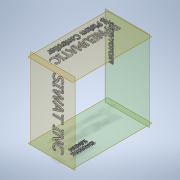
# Autodesk Inventor part: BaseTextYellow
Saved by Autodesk Inventor 2022.2 (Build 262287000, 287)
## iProperties
Created: 2022-01-15
Part Number: BaseTextYellow
Material: Generic
Document SubType Name: Modeling
Designer: siwat
Density: 1 g/cm^3
Appearance: Default
Author: siwat
Autodesk Inventor part; units mm, degrees
(part 1 of 2)
ref_plane "YZ Plane" through (0, 0, 0) normal (1, 0, 0) x (0, 1, 0)
ref_plane "XZ Plane" through (0, 0, 0) normal (0, 1, 0) x (-1, 0, 0)
ref_plane "XY Plane" through (0, 0, 0) normal (0, 0, 1) x (1, 0, 0)
ref_plane "Work Plane1" through (0, 0, 0) normal (0, 0, 1) x (1, 0, 0)
sketch "Sketch1" plane through (0, 0, 0) normal (0, 0, 1) x (1, 0, 0)
  line L0 (54.655, -7.723) -> (54.655, -141.093) construction
  line L1 (54.655, -141.093) -> (34.3574, -141.093) construction
  line L2 (34.3574, -141.093) -> (34.3574, -7.723) construction
  line L3 (34.3574, -7.723) -> (54.655, -7.723) construction
  spline S0 degree 2 poles (34.9775, -14.9442) (34.9775, -12.881) (35.8397, -9.9864) (36.4556, -8.7084) knots 0 0 0 1 2 2 2
  line L4 (36.4556, -8.7084) -> (39.6274, -8.7084)
  line L5 (39.6274, -8.7084) -> (39.6274, -8.8932)
  spline S1 degree 2 poles (39.6274, -8.8932) (38.4572, -10.1403) (37.1639, -13.2967) (37.1639, -14.7594) knots 0 0 0 1 2 2 2
  spline S2 degree 2 poles (37.1639, -14.7594) (37.1639, -16.8535) (38.9037, -18.9936) (40.3357, -18.9936) knots 0 0 0 1 2 2 2
  spline S3 degree 2 poles (40.3357, -18.9936) (41.4751, -18.9936) (42.8916, -17.8697) (43.2457, -16.6533) knots 0 0 0 1 2 2 2
  spline S4 degree 2 poles (43.2457, -16.6533) (43.4921, -15.7757) (43.8308, -14.3129) (44.108, -13.2197) knots 0 0 0 1 2 2 2
  spline S5 degree 2 poles (44.108, -13.2197) (44.3697, -12.2343) (45.155, -10.6792) (45.7862, -10.0787) knots 0 0 0 1 2 2 2
  spline S6 degree 2 poles (45.7862, -10.0787) (46.4175, -9.4936) (48.1112, -8.847) (49.2198, -8.847) knots 0 0 0 1 2 2 2
  spline S7 degree 2 poles (49.2198, -8.847) (51.5294, -8.847) (54.655, -12.4499) (54.655, -15.2368) knots 0 0 0 1 2 2 2
  spline S8 degree 2 poles (54.655, -15.2368) (54.655, -16.8381) (54.0237, -19.6711) (53.4232, -20.8875) knots 0 0 0 1 2 2 2
  line L6 (53.4232, -20.8875) -> (50.4054, -20.8875)
  line L7 (50.4054, -20.8875) -> (50.4054, -20.7027)
  spline S9 degree 2 poles (50.4054, -20.7027) (51.2368, -19.7943) (52.4686, -16.9612) (52.4686, -15.4061) knots 0 0 0 1 2 2 2
  spline S10 degree 2 poles (52.4686, -15.4061) (52.4686, -13.6509) (50.8211, -11.4799) (49.4815, -11.4799) knots 0 0 0 1 2 2 2
  spline S11 degree 2 poles (49.4815, -11.4799) (48.2806, -11.4799) (46.8486, -12.7578) (46.5253, -13.9588) knots 0 0 0 1 2 2 2
  spline S12 degree 2 poles (46.5253, -13.9588) (46.3097, -14.7594) (45.7554, -17.0844) (45.5245, -17.8543) knots 0 0 0 1 2 2 2
  spline S13 degree 2 poles (45.5245, -17.8543) (44.924, -19.8097) (42.5067, -21.6265) (40.736, -21.6265) knots 0 0 0 1 2 2 2
  spline S14 degree 2 poles (40.736, -21.6265) (39.612, -21.6265) (37.4564, -20.7181) (36.702, -19.9021) knots 0 0 0 1 2 2 2
  spline S15 degree 2 poles (36.702, -19.9021) (35.8705, -18.9936) (34.9775, -16.6841) (34.9775, -14.9442) knots 0 0 0 1 2 2 2
  line L8 (35.3162, -30.8186) -> (35.3162, -23.4588)
  line L9 (35.3162, -23.4588) -> (37.2563, -23.4588)
  line L10 (37.2563, -23.4588) -> (37.2563, -25.8761)
  line L11 (37.2563, -25.8761) -> (52.3762, -25.8761)
  line L12 (52.3762, -25.8761) -> (52.3762, -23.4588)
  line L13 (52.3762, -23.4588) -> (54.3162, -23.4588)
  line L14 (54.3162, -23.4588) -> (54.3162, -30.8186)
  line L15 (54.3162, -30.8186) -> (52.3762, -30.8186)
  line L16 (52.3762, -30.8186) -> (52.3762, -28.4013)
  line L17 (52.3762, -28.4013) -> (37.2563, -28.4013)
  line L18 (37.2563, -28.4013) -> (37.2563, -30.8186)
  line L19 (37.2563, -30.8186) -> (35.3162, -30.8186)
  line L20 (54.3162, -55.2384) -> (35.3162, -50.4653)
  line L21 (35.3162, -50.4653) -> (35.3162, -47.6322)
  line L22 (35.3162, -47.6322) -> (51.0828, -43.7676)
  line L23 (51.0828, -43.7676) -> (35.3162, -40.0107)
  line L24 (35.3162, -40.0107) -> (35.3162, -37.2084)
  line L25 (35.3162, -37.2084) -> (54.3162, -32.3583)
  line L26 (54.3162, -32.3583) -> (54.3162, -34.9604)
  line L27 (54.3162, -34.9604) -> (38.565, -38.7789)
  line L28 (38.565, -38.7789) -> (54.3162, -42.5666)
  line L29 (54.3162, -42.5666) -> (54.3162, -45.1379)
  line L30 (54.3162, -45.1379) -> (38.3802, -48.9564)
  line L31 (38.3802, -48.9564) -> (54.3162, -52.7594)
  line L32 (54.3162, -52.7594) -> (54.3162, -55.2384)
  line L33 (35.3162, -55.4539) -> (54.3162, -61.8591)
  line L34 (54.3162, -61.8591) -> (54.3162, -64.9693)
  line L35 (54.3162, -64.9693) -> (35.3162, -71.3745)
  line L36 (35.3162, -71.3745) -> (35.3162, -68.7108)
  line L37 (35.3162, -68.7108) -> (40.6282, -66.9864)
  line L38 (40.6282, -66.9864) -> (40.6282, -59.7343)
  line L39 (40.6282, -59.7343) -> (35.3162, -58.0099)
  line L40 (35.3162, -58.0099) -> (35.3162, -55.4539)
  line L41 (42.7838, -66.2935) -> (51.7295, -63.3526)
  line L42 (51.7295, -63.3526) -> (42.7838, -60.4272)
  line L43 (42.7838, -60.4272) -> (42.7838, -66.2935)
  line L44 (35.3162, -77.6103) -> (52.0683, -77.6103)
  line L45 (52.0683, -77.6103) -> (52.0683, -71.2359)
  line L46 (52.0683, -71.2359) -> (54.3162, -71.2359)
  line L47 (54.3162, -71.2359) -> (54.3162, -86.5099)
  line L48 (54.3162, -86.5099) -> (52.0683, -86.5099)
  line L49 (52.0683, -86.5099) -> (52.0683, -80.1355)
  line L50 (52.0683, -80.1355) -> (35.3162, -80.1355)
  line L51 (35.3162, -80.1355) -> (35.3162, -77.6103)
  line L52 (35.3162, -103.2157) -> (35.3162, -95.8559)
  line L53 (35.3162, -95.8559) -> (37.2563, -95.8559)
  line L54 (37.2563, -95.8559) -> (37.2563, -98.2732)
  line L55 (37.2563, -98.2732) -> (52.3762, -98.2732)
  line L56 (52.3762, -98.2732) -> (52.3762, -95.8559)
  line L57 (52.3762, -95.8559) -> (54.3162, -95.8559)
  line L58 (54.3162, -95.8559) -> (54.3162, -103.2157)
  line L59 (54.3162, -103.2157) -> (52.3762, -103.2157)
  line L60 (52.3762, -103.2157) -> (52.3762, -100.7983)
  line L61 (52.3762, -100.7983) -> (37.2563, -100.7983)
  line L62 (37.2563, -100.7983) -> (37.2563, -103.2157)
  line L63 (37.2563, -103.2157) -> (35.3162, -103.2157)
  line L64 (35.3162, -119.9369) -> (35.3162, -117.1039)
  line L65 (35.3162, -117.1039) -> (51.6987, -108.697)
  line L66 (51.6987, -108.697) -> (35.3162, -108.697)
  line L67 (35.3162, -108.697) -> (35.3162, -106.3413)
  line L68 (35.3162, -106.3413) -> (54.3162, -106.3413)
  line L69 (54.3162, -106.3413) -> (54.3162, -109.9288)
  line L70 (54.3162, -109.9288) -> (39.2733, -117.5812)
  line L71 (39.2733, -117.5812) -> (54.3162, -117.5812)
  line L72 (54.3162, -117.5812) -> (54.3162, -119.9369)
  line L73 (54.3162, -119.9369) -> (35.3162, -119.9369)
  spline S16 degree 2 poles (34.9775, -131.2076) (34.9775, -129.3599) (36.2247, -126.2343) (37.4718, -125.0949) knots 0 0 0 1 2 2 2
  spline S17 degree 2 poles (37.4718, -125.0949) (38.7036, -123.9556) (42.3989, -122.7084) (44.8008, -122.7084) knots 0 0 0 1 2 2 2
  spline S18 degree 2 poles (44.8008, -122.7084) (47.1874, -122.7084) (50.7287, -123.9248) (52.0375, -125.0795) knots 0 0 0 1 2 2 2
  spline S19 degree 2 poles (52.0375, -125.0795) (53.3154, -126.2189) (54.655, -129.3291) (54.655, -131.2538) knots 0 0 0 1 2 2 2
  spline S20 degree 2 poles (54.655, -131.2538) (54.655, -132.2084) (54.3778, -133.8867) (54.1623, -134.5949) knots 0 0 0 1 2 2 2
  spline S21 degree 2 poles (54.1623, -134.5949) (53.9621, -135.2108) (53.3924, -136.4888) (53.0537, -137.1201) knots 0 0 0 1 2 2 2
  line L74 (53.0537, -137.1201) -> (50.005, -137.1201)
  line L75 (50.005, -137.1201) -> (50.005, -136.9199)
  spline S22 degree 2 poles (50.005, -136.9199) (50.313, -136.5812) (51.1752, -135.5342) (51.5909, -134.7797) knots 0 0 0 1 2 2 2
  spline S23 degree 2 poles (51.5909, -134.7797) (51.9913, -134.056) (52.4994, -132.347) (52.4994, -131.2384) knots 0 0 0 1 2 2 2
  spline S24 degree 2 poles (52.4994, -131.2384) (52.4994, -130.022) (51.4986, -127.851) (50.5439, -127.035) knots 0 0 0 1 2 2 2
  spline S25 degree 2 poles (50.5439, -127.035) (49.5739, -126.2343) (46.6331, -125.3413) (44.8008, -125.3413) knots 0 0 0 1 2 2 2
  spline S26 degree 2 poles (44.8008, -125.3413) (42.8454, -125.3413) (40.0277, -126.2805) (39.0577, -127.0966) knots 0 0 0 1 2 2 2
  spline S27 degree 2 poles (39.0577, -127.0966) (38.1185, -127.8972) (37.1639, -130.0374) (37.1639, -131.2384) knots 0 0 0 1 2 2 2
  spline S28 degree 2 poles (37.1639, -131.2384) (37.1639, -132.3316) (37.7028, -134.1946) (38.1031, -134.9183) knots 0 0 0 1 2 2 2
  spline S29 degree 2 poles (38.1031, -134.9183) (38.5034, -135.6111) (39.3349, -136.6428) (39.6274, -136.9353) knots 0 0 0 1 2 2 2
  line L76 (39.6274, -136.9353) -> (39.6274, -137.1201)
  line L77 (39.6274, -137.1201) -> (36.6096, -137.1201)
  spline S30 degree 2 poles (36.6096, -137.1201) (36.317, -136.4888) (35.7781, -135.3802) (35.5318, -134.5949) knots 0 0 0 1 2 2 2
  spline S31 degree 2 poles (35.5318, -134.5949) (35.2546, -133.7635) (34.9775, -132.347) (34.9775, -131.2076) knots 0 0 0 1 2 2 2
  point P0 (0, 0)
  constraints: 2 other
extrude "Extrusion1" add sketch "Sketch1" against normal blind 2
ref_plane "Work Plane2" through (0, 0, -142.4319) normal (0.0000018, 1, 0) x (0.0015858, 0, 0.9999987)
sketch "Sketch2" plane through (0, 0, -142.4319) normal (0.0000018, 1, 0) x (0.0015858, 0, 0.9999987)
  line L0 (22.3492, 32.6802) -> (316.1985, 32.6802) construction
  line L1 (316.1985, 32.6802) -> (316.1985, 7.1194) construction
  line L2 (316.1985, 7.1194) -> (22.3492, 7.1194) construction
  line L3 (22.3492, 7.1194) -> (22.3492, 32.6802) construction
  line L4 (22.2144, 12.4409) -> (316.0637, 12.4409) construction
  line L5 (316.0637, 12.4409) -> (316.0637, -3.1912) construction
  line L6 (316.0637, -3.1912) -> (22.2144, -3.1912) construction
  line L7 (22.2144, -3.1912) -> (22.2144, 12.4409) construction
  line L8 (10.9639, 9.125) -> (10.9639, 34.4309) construction
  line L9 (10.9639, 34.4309) -> (304.8132, 34.4309) construction
  line L10 (304.8132, 34.4309) -> (304.8132, 9.125) construction
  line L11 (304.8132, 9.125) -> (10.9639, 9.125) construction
  spline S0 degree 2 poles (19.8618, 29.4228) (19.8618, 28.0533) (18.7516, 25.8491) (17.8197, 25.2332) knots 0 0 0 1 2 2 2
  spline S1 degree 2 poles (17.8197, 25.2332) (17.0579, 24.7551) (15.4939, 24.4309) (14.2784, 24.4309) knots 0 0 0 1 2 2 2
  line L12 (14.2784, 24.4309) -> (11.9769, 24.4309)
  line L13 (11.9769, 24.4309) -> (11.9769, 34.4309)
  line L14 (11.9769, 34.4309) -> (14.254, 34.4309)
  spline S2 degree 2 poles (14.254, 34.4309) (15.6641, 34.4309) (17.2686, 34.0096) (17.8359, 33.6368) knots 0 0 0 1 2 2 2
  spline S3 degree 2 poles (17.8359, 33.6368) (18.8002, 32.9966) (19.8618, 30.8815) (19.8618, 29.4228) knots 0 0 0 1 2 2 2
  spline S4 degree 2 poles (18.4761, 29.439) (18.4761, 30.5898) (17.7143, 32.2186) (16.9607, 32.6805) knots 0 0 0 1 2 2 2
  spline S5 degree 2 poles (16.9607, 32.6805) (16.4258, 32.9966) (15.2184, 33.2802) (14.3189, 33.2802) knots 0 0 0 1 2 2 2
  line L15 (14.3189, 33.2802) -> (13.3059, 33.2802)
  line L16 (13.3059, 33.2802) -> (13.3059, 25.5817)
  line L17 (13.3059, 25.5817) -> (14.3189, 25.5817)
  spline S6 degree 2 poles (14.3189, 25.5817) (15.2022, 25.5817) (16.5393, 25.8653) (17.0823, 26.2462) knots 0 0 0 1 2 2 2
  spline S7 degree 2 poles (17.0823, 26.2462) (17.7792, 26.7162) (18.4761, 28.2721) (18.4761, 29.439) knots 0 0 0 1 2 2 2
  line L18 (17.8602, 12.4309) -> (11.6933, 12.4309)
  line L19 (11.6933, 12.4309) -> (11.6933, 13.8491)
  spline S8 degree 2 poles (11.6933, 13.8491) (12.3578, 14.4731) (13.5409, 15.6319) (14.1082, 16.2559) knots 0 0 0 1 2 2 2
  spline S9 degree 2 poles (14.1082, 16.2559) (15.2508, 17.512) (16.0855, 19.0193) (16.0855, 19.8215) knots 0 0 0 1 2 2 2
  spline S10 degree 2 poles (16.0855, 19.8215) (16.0855, 20.2429) (15.8262, 20.875) (15.5912, 21.0776) knots 0 0 0 1 2 2 2
  spline S11 degree 2 poles (15.5912, 21.0776) (15.3562, 21.2802) (14.7403, 21.4828) (14.3675, 21.4828) knots 0 0 0 1 2 2 2
  spline S12 degree 2 poles (14.3675, 21.4828) (14.0109, 21.4828) (13.2816, 21.3045) (12.9493, 21.1668) knots 0 0 0 1 2 2 2
  spline S13 degree 2 poles (12.9493, 21.1668) (12.6657, 21.0533) (12.139, 20.7292) (11.9769, 20.6157) knots 0 0 0 1 2 2 2
  line L20 (11.9769, 20.6157) -> (11.904, 20.6157)
  line L21 (11.904, 20.6157) -> (11.904, 22.042)
  spline S14 degree 2 poles (11.904, 22.042) (12.3173, 22.2446) (13.8002, 22.6416) (14.4647, 22.6416) knots 0 0 0 1 2 2 2
  spline S15 degree 2 poles (14.4647, 22.6416) (15.8667, 22.6416) (17.4469, 21.1587) (17.4469, 19.8945) knots 0 0 0 1 2 2 2
  spline S16 degree 2 poles (17.4469, 19.8945) (17.4469, 19.3029) (17.1714, 18.3143) (16.9283, 17.8929) knots 0 0 0 1 2 2 2
  spline S17 degree 2 poles (16.9283, 17.8929) (16.6852, 17.4553) (15.9801, 16.5963) (15.5912, 16.183) knots 0 0 0 1 2 2 2
  spline S18 degree 2 poles (15.5912, 16.183) (14.9591, 15.4942) (13.4113, 14.0193) (12.9493, 13.5898) knots 0 0 0 1 2 2 2
  line L22 (12.9493, 13.5898) -> (17.8602, 13.5898)
  line L23 (17.8602, 13.5898) -> (17.8602, 12.4309)
  spline S19 degree 2 poles (14.7646, 0.2527) (13.6787, 0.2527) (12.1552, 0.7065) (11.4826, 1.0306) knots 0 0 0 1 2 2 2
  line L24 (11.4826, 1.0306) -> (11.4826, 2.7)
  line L25 (11.4826, 2.7) -> (11.5798, 2.7)
  spline S20 degree 2 poles (11.5798, 2.7) (12.2362, 2.0841) (13.8975, 1.4034) (14.6673, 1.4034) knots 0 0 0 1 2 2 2
  spline S21 degree 2 poles (14.6673, 1.4034) (15.7694, 1.4034) (16.8959, 2.3191) (16.8959, 3.0728) knots 0 0 0 1 2 2 2
  spline S22 degree 2 poles (16.8959, 3.0728) (16.8959, 3.6724) (16.3043, 4.418) (15.6641, 4.6044) knots 0 0 0 1 2 2 2
  spline S23 degree 2 poles (15.6641, 4.6044) (15.2022, 4.734) (14.4323, 4.9123) (13.857, 5.0582) knots 0 0 0 1 2 2 2
  spline S24 degree 2 poles (13.857, 5.0582) (13.3383, 5.1959) (12.5199, 5.6092) (12.2038, 5.9415) knots 0 0 0 1 2 2 2
  spline S25 degree 2 poles (12.2038, 5.9415) (11.8959, 6.2737) (11.5555, 7.1651) (11.5555, 7.7486) knots 0 0 0 1 2 2 2
  spline S26 degree 2 poles (11.5555, 7.7486) (11.5555, 8.9642) (13.4518, 10.6092) (14.9186, 10.6092) knots 0 0 0 1 2 2 2
  spline S27 degree 2 poles (14.9186, 10.6092) (15.7613, 10.6092) (17.2524, 10.277) (17.8926, 9.9609) knots 0 0 0 1 2 2 2
  line L26 (17.8926, 9.9609) -> (17.8926, 8.3726)
  line L27 (17.8926, 8.3726) -> (17.7954, 8.3726)
  spline S28 degree 2 poles (17.7954, 8.3726) (17.3173, 8.8102) (15.8262, 9.4585) (15.0077, 9.4585) knots 0 0 0 1 2 2 2
  spline S29 degree 2 poles (15.0077, 9.4585) (14.0839, 9.4585) (12.9412, 8.5914) (12.9412, 7.8864) knots 0 0 0 1 2 2 2
  spline S30 degree 2 poles (12.9412, 7.8864) (12.9412, 7.2543) (13.6139, 6.5006) (14.2459, 6.3305) knots 0 0 0 1 2 2 2
  spline S31 degree 2 poles (14.2459, 6.3305) (14.6673, 6.217) (15.891, 5.9253) (16.2962, 5.8037) knots 0 0 0 1 2 2 2
  spline S32 degree 2 poles (16.2962, 5.8037) (17.3254, 5.4877) (18.2816, 4.2154) (18.2816, 3.2835) knots 0 0 0 1 2 2 2
  spline S33 degree 2 poles (18.2816, 3.2835) (18.2816, 2.6919) (17.8035, 1.5574) (17.374, 1.1603) knots 0 0 0 1 2 2 2
  spline S34 degree 2 poles (17.374, 1.1603) (16.8959, 0.7227) (15.6803, 0.2527) (14.7646, 0.2527) knots 0 0 0 1 2 2 2
  spline S35 degree 2 poles (33.35, 27.8909) (33.35, 26.9184) (32.6571, 25.168) (32.0372, 24.5602) knots 0 0 0 1 2 2 2
  spline S36 degree 2 poles (32.0372, 24.5602) (31.2592, 23.7944) (29.1563, 23.0043) (27.5518, 23.0043) knots 0 0 0 1 2 2 2
  line L28 (27.5518, 23.0043) -> (25.8621, 23.0043)
  line L29 (25.8621, 23.0043) -> (25.8621, 17.4127)
  line L30 (25.8621, 17.4127) -> (23.8686, 17.4127)
  line L31 (23.8686, 17.4127) -> (23.8686, 32.4127)
  line L32 (23.8686, 32.4127) -> (27.6369, 32.4127)
  spline S37 degree 2 poles (27.6369, 32.4127) (28.974, 32.4127) (30.8459, 31.9751) (31.5631, 31.4768) knots 0 0 0 1 2 2 2
  spline S38 degree 2 poles (31.5631, 31.4768) (32.4019, 30.9055) (33.35, 29.1429) (33.35, 27.8909) knots 0 0 0 1 2 2 2
  spline S39 degree 2 poles (31.2714, 27.8301) (31.2714, 28.608) (30.7365, 29.7507) (30.1895, 30.1153) knots 0 0 0 1 2 2 2
  spline S40 degree 2 poles (30.1895, 30.1153) (29.7155, 30.4314) (28.4513, 30.6867) (27.5153, 30.6867) knots 0 0 0 1 2 2 2
  line L33 (27.5153, 30.6867) -> (25.8621, 30.6867)
  line L34 (25.8621, 30.6867) -> (25.8621, 24.7061)
  line L35 (25.8621, 24.7061) -> (27.2236, 24.7061)
  spline S41 degree 2 poles (27.2236, 24.7061) (28.4391, 24.7061) (29.9343, 25.0951) (30.4205, 25.6056) knots 0 0 0 1 2 2 2
  spline S42 degree 2 poles (30.4205, 25.6056) (30.8702, 26.0554) (31.2714, 27.1129) (31.2714, 27.8301) knots 0 0 0 1 2 2 2
  line L36 (45.9796, 17.4127) -> (43.743, 17.4127)
  line L37 (43.743, 17.4127) -> (37.1061, 30.3463)
  line L38 (37.1061, 30.3463) -> (37.1061, 17.4127)
  line L39 (37.1061, 17.4127) -> (35.2463, 17.4127)
  line L40 (35.2463, 17.4127) -> (35.2463, 32.4127)
  line L41 (35.2463, 32.4127) -> (38.0785, 32.4127)
  line L42 (38.0785, 32.4127) -> (44.1198, 20.5367)
  line L43 (44.1198, 20.5367) -> (44.1198, 32.4127)
  line L44 (44.1198, 32.4127) -> (45.9796, 32.4127)
  line L45 (45.9796, 32.4127) -> (45.9796, 17.4127)
  line L46 (49.0185, 17.4127) -> (49.0185, 32.4127)
  line L47 (49.0185, 32.4127) -> (58.4027, 32.4127)
  line L48 (58.4027, 32.4127) -> (58.4027, 30.638)
  line L49 (58.4027, 30.638) -> (51.0121, 30.638)
  line L50 (51.0121, 30.638) -> (51.0121, 26.5294)
  line L51 (51.0121, 26.5294) -> (57.9043, 26.5294)
  line L52 (57.9043, 26.5294) -> (57.9043, 24.7547)
  line L53 (57.9043, 24.7547) -> (51.0121, 24.7547)
  line L54 (51.0121, 24.7547) -> (51.0121, 19.1875)
  line L55 (51.0121, 19.1875) -> (58.4027, 19.1875)
  line L56 (58.4027, 19.1875) -> (58.4027, 17.4127)
  line L57 (58.4027, 17.4127) -> (49.0185, 17.4127)
  spline S43 degree 2 poles (65.8297, 17.0967) (64.5048, 17.0967) (62.5356, 17.7896) (61.8427, 18.4824) knots 0 0 0 1 2 2 2
  spline S44 degree 2 poles (61.8427, 18.4824) (61.0526, 19.2604) (60.4083, 21.4484) (60.4083, 23.0529) knots 0 0 0 1 2 2 2
  line L58 (60.4083, 23.0529) -> (60.4083, 32.4127)
  line L59 (60.4083, 32.4127) -> (62.4019, 32.4127)
  line L60 (62.4019, 32.4127) -> (62.4019, 23.0529)
  spline S45 degree 2 poles (62.4019, 23.0529) (62.4019, 22.0076) (62.6693, 20.5975) (63.0461, 20.0262) knots 0 0 0 1 2 2 2
  spline S46 degree 2 poles (63.0461, 20.0262) (63.4472, 19.4184) (64.833, 18.7985) (65.8297, 18.7985) knots 0 0 0 1 2 2 2
  spline S47 degree 2 poles (65.8297, 18.7985) (66.7657, 18.7985) (68.2244, 19.4184) (68.6255, 20.0262) knots 0 0 0 1 2 2 2
  spline S48 degree 2 poles (68.6255, 20.0262) (69.0023, 20.5975) (69.2698, 21.9954) (69.2698, 23.0043) knots 0 0 0 1 2 2 2
  line L61 (69.2698, 23.0043) -> (69.2698, 32.4127)
  line L62 (69.2698, 32.4127) -> (71.2633, 32.4127)
  line L63 (71.2633, 32.4127) -> (71.2633, 23.0529)
  spline S49 degree 2 poles (71.2633, 23.0529) (71.2633, 21.4849) (70.6312, 19.2482) (69.8289, 18.4824) knots 0 0 0 1 2 2 2
  spline S50 degree 2 poles (69.8289, 18.4824) (69.1117, 17.7774) (67.2155, 17.0967) (65.8297, 17.0967) knots 0 0 0 1 2 2 2
  line L64 (86.9805, 17.4127) -> (84.9869, 17.4127)
  line L65 (84.9869, 17.4127) -> (84.9869, 30.3341)
  line L66 (84.9869, 30.3341) -> (81.0728, 21.5456)
  line L67 (81.0728, 21.5456) -> (79.8573, 21.5456)
  line L68 (79.8573, 21.5456) -> (75.9796, 30.3341)
  line L69 (75.9796, 30.3341) -> (75.9796, 17.4127)
  line L70 (75.9796, 17.4127) -> (74.1198, 17.4127)
  line L71 (74.1198, 17.4127) -> (74.1198, 32.4127)
  line L72 (74.1198, 32.4127) -> (76.8427, 32.4127)
  line L73 (76.8427, 32.4127) -> (80.5866, 24.0619)
  line L74 (80.5866, 24.0619) -> (84.209, 32.4127)
  line L75 (84.209, 32.4127) -> (86.9805, 32.4127)
  line L76 (86.9805, 32.4127) -> (86.9805, 17.4127)
  line L77 (88.4027, 17.4127) -> (93.4594, 32.4127)
  line L78 (93.4594, 32.4127) -> (95.9148, 32.4127)
  line L79 (95.9148, 32.4127) -> (100.9715, 17.4127)
  line L80 (100.9715, 17.4127) -> (98.8686, 17.4127)
  line L81 (98.8686, 17.4127) -> (97.5072, 21.6064)
  line L82 (97.5072, 21.6064) -> (91.7819, 21.6064)
  line L83 (91.7819, 21.6064) -> (90.4205, 17.4127)
  line L84 (90.4205, 17.4127) -> (88.4027, 17.4127)
  line L85 (96.9602, 23.3082) -> (94.6385, 30.3706)
  line L86 (94.6385, 30.3706) -> (92.3289, 23.3082)
  line L87 (92.3289, 23.3082) -> (96.9602, 23.3082)
  line L88 (105.8946, 17.4127) -> (105.8946, 30.638)
  line L89 (105.8946, 30.638) -> (100.8621, 30.638)
  line L90 (100.8621, 30.638) -> (100.8621, 32.4127)
  line L91 (100.8621, 32.4127) -> (112.9205, 32.4127)
  line L92 (112.9205, 32.4127) -> (112.9205, 30.638)
  line L93 (112.9205, 30.638) -> (107.8881, 30.638)
  line L94 (107.8881, 30.638) -> (107.8881, 17.4127)
  line L95 (107.8881, 17.4127) -> (105.8946, 17.4127)
  line L96 (119.6668, 17.4127) -> (113.8565, 17.4127)
  line L97 (113.8565, 17.4127) -> (113.8565, 18.9444)
  line L98 (113.8565, 18.9444) -> (115.7649, 18.9444)
  line L99 (115.7649, 18.9444) -> (115.7649, 30.8811)
  line L100 (115.7649, 30.8811) -> (113.8565, 30.8811)
  line L101 (113.8565, 30.8811) -> (113.8565, 32.4127)
  line L102 (113.8565, 32.4127) -> (119.6668, 32.4127)
  line L103 (119.6668, 32.4127) -> (119.6668, 30.8811)
  line L104 (119.6668, 30.8811) -> (117.7584, 30.8811)
  line L105 (117.7584, 30.8811) -> (117.7584, 18.9444)
  line L106 (117.7584, 18.9444) -> (119.6668, 18.9444)
  line L107 (119.6668, 18.9444) -> (119.6668, 17.4127)
  spline S51 degree 2 poles (127.9934, 17.1453) (126.5348, 17.1453) (124.0672, 18.1299) (123.1677, 19.1145) knots 0 0 0 1 2 2 2
  spline S52 degree 2 poles (123.1677, 19.1145) (122.2681, 20.087) (121.2835, 23.0043) (121.2835, 24.9006) knots 0 0 0 1 2 2 2
  spline S53 degree 2 poles (121.2835, 24.9006) (121.2835, 26.7847) (122.2438, 29.5805) (123.1555, 30.6137) knots 0 0 0 1 2 2 2
  spline S54 degree 2 poles (123.1555, 30.6137) (124.055, 31.6226) (126.5104, 32.6802) (128.0299, 32.6802) knots 0 0 0 1 2 2 2
  spline S55 degree 2 poles (128.0299, 32.6802) (128.7835, 32.6802) (130.1085, 32.4614) (130.6677, 32.2912) knots 0 0 0 1 2 2 2
  spline S56 degree 2 poles (130.6677, 32.2912) (131.1539, 32.1332) (132.1628, 31.6834) (132.6612, 31.416) knots 0 0 0 1 2 2 2
  line L108 (132.6612, 31.416) -> (132.6612, 29.0092)
  line L109 (132.6612, 29.0092) -> (132.5031, 29.0092)
  spline S57 degree 2 poles (132.5031, 29.0092) (132.2357, 29.2523) (131.4091, 29.933) (130.8135, 30.2612) knots 0 0 0 1 2 2 2
  spline S58 degree 2 poles (130.8135, 30.2612) (130.2422, 30.5773) (128.8929, 30.9784) (128.0177, 30.9784) knots 0 0 0 1 2 2 2
  spline S59 degree 2 poles (128.0177, 30.9784) (127.0574, 30.9784) (125.3435, 30.1883) (124.6993, 29.4346) knots 0 0 0 1 2 2 2
  spline S60 degree 2 poles (124.6993, 29.4346) (124.0672, 28.6688) (123.3621, 26.3471) (123.3621, 24.9006) knots 0 0 0 1 2 2 2
  spline S61 degree 2 poles (123.3621, 24.9006) (123.3621, 23.3568) (124.1036, 21.1324) (124.7479, 20.3666) knots 0 0 0 1 2 2 2
  spline S62 degree 2 poles (124.7479, 20.3666) (125.38, 19.6251) (127.0696, 18.8714) (128.0177, 18.8714) knots 0 0 0 1 2 2 2
  spline S63 degree 2 poles (128.0177, 18.8714) (128.8808, 18.8714) (130.3516, 19.2969) (130.9229, 19.6129) knots 0 0 0 1 2 2 2
  spline S64 degree 2 poles (130.9229, 19.6129) (131.4699, 19.929) (132.2843, 20.5854) (132.5153, 20.8163) knots 0 0 0 1 2 2 2
  line L110 (132.5153, 20.8163) -> (132.6612, 20.8163)
  line L111 (132.6612, 20.8163) -> (132.6612, 18.4338)
  spline S65 degree 2 poles (132.6612, 18.4338) (132.1628, 18.2029) (131.2876, 17.7774) (130.6677, 17.5829) knots 0 0 0 1 2 2 2
  spline S66 degree 2 poles (130.6677, 17.5829) (130.0113, 17.3641) (128.8929, 17.1453) (127.9934, 17.1453) knots 0 0 0 1 2 2 2
  spline S67 degree 2 poles (29.5483, 8.9806) (29.5483, 8.3323) (29.0864, 7.1654) (28.6731, 6.7602) knots 0 0 0 1 2 2 2
  spline S68 degree 2 poles (28.6731, 6.7602) (28.1545, 6.2497) (26.7525, 5.7229) (25.6828, 5.7229) knots 0 0 0 1 2 2 2
  line L112 (25.6828, 5.7229) -> (24.5564, 5.7229)
  line L113 (24.5564, 5.7229) -> (24.5564, 1.9952)
  line L114 (24.5564, 1.9952) -> (23.2274, 1.9952)
  line L115 (23.2274, 1.9952) -> (23.2274, 11.9952)
  line L116 (23.2274, 11.9952) -> (25.7395, 11.9952)
  spline S69 degree 2 poles (25.7395, 11.9952) (26.631, 11.9952) (27.8789, 11.7035) (28.357, 11.3712) knots 0 0 0 1 2 2 2
  spline S70 degree 2 poles (28.357, 11.3712) (28.9162, 10.9904) (29.5483, 9.8153) (29.5483, 8.9806) knots 0 0 0 1 2 2 2
  spline S71 degree 2 poles (28.1626, 8.9401) (28.1626, 9.4587) (27.806, 10.2205) (27.4413, 10.4636) knots 0 0 0 1 2 2 2
  spline S72 degree 2 poles (27.4413, 10.4636) (27.1253, 10.6743) (26.2825, 10.8445) (25.6585, 10.8445) knots 0 0 0 1 2 2 2
  line L117 (25.6585, 10.8445) -> (24.5564, 10.8445)
  line L118 (24.5564, 10.8445) -> (24.5564, 6.8575)
  line L119 (24.5564, 6.8575) -> (25.464, 6.8575)
  spline S73 degree 2 poles (25.464, 6.8575) (26.2744, 6.8575) (27.2711, 7.1168) (27.5953, 7.4571) knots 0 0 0 1 2 2 2
  spline S74 degree 2 poles (27.5953, 7.4571) (27.8951, 7.757) (28.1626, 8.462) (28.1626, 8.9401) knots 0 0 0 1 2 2 2
  line L120 (32.0037, 1.9952) -> (30.7395, 1.9952)
  line L121 (30.7395, 1.9952) -> (30.7395, 9.4993)
  line L122 (30.7395, 9.4993) -> (32.0037, 9.4993)
  line L123 (32.0037, 9.4993) -> (32.0037, 1.9952)
  line L124 (32.0929, 10.7472) -> (30.6585, 10.7472)
  line L125 (30.6585, 10.7472) -> (30.6585, 12.06)
  line L126 (30.6585, 12.06) -> (32.0929, 12.06)
  line L127 (32.0929, 12.06) -> (32.0929, 10.7472)
  spline S75 degree 2 poles (35.8854, 1.8169) (35.1318, 1.8169) (33.8271, 2.2221) (33.3976, 2.449) knots 0 0 0 1 2 2 2
  line L128 (33.3976, 2.449) -> (33.3976, 3.8672)
  line L129 (33.3976, 3.8672) -> (33.4624, 3.8672)
  spline S76 degree 2 poles (33.4624, 3.8672) (33.6245, 3.7375) (34.0621, 3.4296) (34.4267, 3.2594) knots 0 0 0 1 2 2 2
  spline S77 degree 2 poles (34.4267, 3.2594) (34.7428, 3.1054) (35.5207, 2.8785) (35.934, 2.8785) knots 0 0 0 1 2 2 2
  spline S78 degree 2 poles (35.934, 2.8785) (36.2339, 2.8785) (36.9227, 3.0163) (37.0848, 3.1297) knots 0 0 0 1 2 2 2
  spline S79 degree 2 poles (37.0848, 3.1297) (37.3198, 3.2837) (37.5305, 3.6322) (37.5305, 3.9887) knots 0 0 0 1 2 2 2
  spline S80 degree 2 poles (37.5305, 3.9887) (37.5305, 4.4344) (37.0442, 4.8964) (36.4203, 5.0503) knots 0 0 0 1 2 2 2
  spline S81 degree 2 poles (36.4203, 5.0503) (36.1771, 5.107) (35.3992, 5.2691) (35.0669, 5.3583) knots 0 0 0 1 2 2 2
  spline S82 degree 2 poles (35.0669, 5.3583) (34.2079, 5.6095) (33.43, 6.6468) (33.43, 7.3842) knots 0 0 0 1 2 2 2
  spline S83 degree 2 poles (33.43, 7.3842) (33.43, 8.4053) (34.9616, 9.6776) (36.2258, 9.6776) knots 0 0 0 1 2 2 2
  spline S84 degree 2 poles (36.2258, 9.6776) (36.8498, 9.6776) (38.1139, 9.3696) (38.5434, 9.1346) knots 0 0 0 1 2 2 2
  line L130 (38.5434, 9.1346) -> (38.5434, 7.7813)
  line L131 (38.5434, 7.7813) -> (38.4786, 7.7813)
  spline S85 degree 2 poles (38.4786, 7.7813) (37.9924, 8.1703) (36.8092, 8.616) (36.2015, 8.616) knots 0 0 0 1 2 2 2
  spline S86 degree 2 poles (36.2015, 8.616) (35.5775, 8.616) (34.7185, 8.0892) (34.7185, 7.5625) knots 0 0 0 1 2 2 2
  spline S87 degree 2 poles (34.7185, 7.5625) (34.7185, 7.0844) (35.229, 6.6224) (35.7963, 6.4766) knots 0 0 0 1 2 2 2
  spline S88 degree 2 poles (35.7963, 6.4766) (36.0718, 6.4036) (36.7687, 6.2578) (37.1496, 6.1686) knots 0 0 0 1 2 2 2
  spline S89 degree 2 poles (37.1496, 6.1686) (37.9762, 5.9579) (38.819, 4.9936) (38.819, 4.1589) knots 0 0 0 1 2 2 2
  spline S90 degree 2 poles (38.819, 4.1589) (38.819, 3.6727) (38.4381, 2.8137) (38.0653, 2.4976) knots 0 0 0 1 2 2 2
  spline S91 degree 2 poles (38.0653, 2.4976) (37.6682, 2.1654) (36.6553, 1.8169) (35.8854, 1.8169) knots 0 0 0 1 2 2 2
  spline S92 degree 2 poles (42.263, 1.8493) (41.2339, 1.8493) (40.075, 3.0244) (40.075, 4.2967) knots 0 0 0 1 2 2 2
  line L132 (40.075, 4.2967) -> (40.075, 8.4539)
  line L133 (40.075, 8.4539) -> (39.2241, 8.4539)
  line L134 (39.2241, 8.4539) -> (39.2241, 9.4993)
  line L135 (39.2241, 9.4993) -> (40.075, 9.4993)
  line L136 (40.075, 9.4993) -> (40.075, 11.6549)
  line L137 (40.075, 11.6549) -> (41.3392, 11.6549)
  line L138 (41.3392, 11.6549) -> (41.3392, 9.4993)
  line L139 (41.3392, 9.4993) -> (43.665, 9.4993)
  line L140 (43.665, 9.4993) -> (43.665, 8.4539)
  line L141 (43.665, 8.4539) -> (41.3392, 8.4539)
  line L142 (41.3392, 8.4539) -> (41.3392, 4.8801)
  spline S93 degree 2 poles (41.3392, 4.8801) (41.3392, 4.3129) (41.3797, 3.6889) (41.5175, 3.4215) knots 0 0 0 1 2 2 2
  spline S94 degree 2 poles (41.5175, 3.4215) (41.631, 3.1865) (42.1415, 2.9515) (42.5791, 2.9515) knots 0 0 0 1 2 2 2
  spline S95 degree 2 poles (42.5791, 2.9515) (42.887, 2.9515) (43.4624, 3.1378) (43.5921, 3.1946) knots 0 0 0 1 2 2 2
  line L143 (43.5921, 3.1946) -> (43.665, 3.1946)
  line L144 (43.665, 3.1946) -> (43.665, 2.06)
  spline S96 degree 2 poles (43.665, 2.06) (43.3084, 1.9628) (42.5791, 1.8493) (42.263, 1.8493) knots 0 0 0 1 2 2 2
  spline S97 degree 2 poles (50.7639, 5.7472) (50.7639, 3.851) (48.9405, 1.7845) (47.417, 1.7845) knots 0 0 0 1 2 2 2
  spline S98 degree 2 poles (47.417, 1.7845) (45.853, 1.7845) (44.0621, 3.9158) (44.0621, 5.7472) knots 0 0 0 1 2 2 2
  spline S99 degree 2 poles (44.0621, 5.7472) (44.0621, 7.6273) (45.9097, 9.71) (47.417, 9.71) knots 0 0 0 1 2 2 2
  spline S100 degree 2 poles (47.417, 9.71) (48.9405, 9.71) (50.7639, 7.6354) (50.7639, 5.7472) knots 0 0 0 1 2 2 2
  spline S101 degree 2 poles (49.4592, 5.7472) (49.4592, 7.2059) (48.3976, 8.6241) (47.417, 8.6241) knots 0 0 0 1 2 2 2
  spline S102 degree 2 poles (47.417, 8.6241) (46.4365, 8.6241) (45.3668, 7.2059) (45.3668, 5.7472) knots 0 0 0 1 2 2 2
  spline S103 degree 2 poles (45.3668, 5.7472) (45.3668, 4.3291) (46.4365, 2.8704) (47.417, 2.8704) knots 0 0 0 1 2 2 2
  spline S104 degree 2 poles (47.417, 2.8704) (48.3895, 2.8704) (49.4592, 4.3048) (49.4592, 5.7472) knots 0 0 0 1 2 2 2
  line L145 (57.9519, 1.9952) -> (56.6877, 1.9952)
  line L146 (56.6877, 1.9952) -> (56.6877, 6.274)
  spline S105 degree 2 poles (56.6877, 6.274) (56.6877, 6.7926) (56.5904, 7.684) (56.4446, 7.9515) knots 0 0 0 1 2 2 2
  spline S106 degree 2 poles (56.4446, 7.9515) (56.2906, 8.2351) (55.7395, 8.5106) (55.2695, 8.5106) knots 0 0 0 1 2 2 2
  spline S107 degree 2 poles (55.2695, 8.5106) (54.7995, 8.5106) (53.8028, 8.0082) (53.3246, 7.603) knots 0 0 0 1 2 2 2
  line L147 (53.3246, 7.603) -> (53.3246, 1.9952)
  line L148 (53.3246, 1.9952) -> (52.0605, 1.9952)
  line L149 (52.0605, 1.9952) -> (52.0605, 9.4993)
  line L150 (52.0605, 9.4993) -> (53.3246, 9.4993)
  line L151 (53.3246, 9.4993) -> (53.3246, 8.6646)
  spline S108 degree 2 poles (53.3246, 8.6646) (53.8919, 9.1751) (54.9859, 9.71) (55.6018, 9.71) knots 0 0 0 1 2 2 2
  spline S109 degree 2 poles (55.6018, 9.71) (56.7039, 9.71) (57.9519, 8.2513) (57.9519, 6.8656) knots 0 0 0 1 2 2 2
  line L152 (57.9519, 6.8656) -> (57.9519, 1.9952)
  spline S110 degree 2 poles (68.0248, 1.8169) (67.0523, 1.8169) (65.4073, 2.4733) (64.8076, 3.1297) knots 0 0 0 1 2 2 2
  spline S111 degree 2 poles (64.8076, 3.1297) (64.2079, 3.778) (63.5515, 5.7229) (63.5515, 6.9871) knots 0 0 0 1 2 2 2
  spline S112 degree 2 poles (63.5515, 6.9871) (63.5515, 8.2432) (64.1917, 10.107) (64.7995, 10.7959) knots 0 0 0 1 2 2 2
  spline S113 degree 2 poles (64.7995, 10.7959) (65.3992, 11.4685) (67.0361, 12.1735) (68.0491, 12.1735) knots 0 0 0 1 2 2 2
  spline S114 degree 2 poles (68.0491, 12.1735) (68.5515, 12.1735) (69.4348, 12.0276) (69.8076, 11.9142) knots 0 0 0 1 2 2 2
  spline S115 degree 2 poles (69.8076, 11.9142) (70.1318, 11.8088) (70.8044, 11.509) (71.1366, 11.3307) knots 0 0 0 1 2 2 2
  line L153 (71.1366, 11.3307) -> (71.1366, 9.7262)
  line L154 (71.1366, 9.7262) -> (71.0313, 9.7262)
  spline S116 degree 2 poles (71.0313, 9.7262) (70.853, 9.8882) (70.3019, 10.3421) (69.9049, 10.5609) knots 0 0 0 1 2 2 2
  spline S117 degree 2 poles (69.9049, 10.5609) (69.524, 10.7716) (68.6245, 11.039) (68.041, 11.039) knots 0 0 0 1 2 2 2
  spline S118 degree 2 poles (68.041, 11.039) (67.4008, 11.039) (66.2582, 10.5122) (65.8287, 10.0098) knots 0 0 0 1 2 2 2
  spline S119 degree 2 poles (65.8287, 10.0098) (65.4073, 9.4993) (64.9373, 7.9515) (64.9373, 6.9871) knots 0 0 0 1 2 2 2
  spline S120 degree 2 poles (64.9373, 6.9871) (64.9373, 5.9579) (65.4316, 4.475) (65.8611, 3.9644) knots 0 0 0 1 2 2 2
  spline S121 degree 2 poles (65.8611, 3.9644) (66.2825, 3.4701) (67.4089, 2.9677) (68.041, 2.9677) knots 0 0 0 1 2 2 2
  spline S122 degree 2 poles (68.041, 2.9677) (68.6164, 2.9677) (69.5969, 3.2513) (69.9778, 3.462) knots 0 0 0 1 2 2 2
  spline S123 degree 2 poles (69.9778, 3.462) (70.3425, 3.6727) (70.8854, 4.1103) (71.0394, 4.2643) knots 0 0 0 1 2 2 2
  line L155 (71.0394, 4.2643) -> (71.1366, 4.2643)
  line L156 (71.1366, 4.2643) -> (71.1366, 2.6759)
  spline S124 degree 2 poles (71.1366, 2.6759) (70.8044, 2.522) (70.2209, 2.2383) (69.8076, 2.1087) knots 0 0 0 1 2 2 2
  spline S125 degree 2 poles (69.8076, 2.1087) (69.37, 1.9628) (68.6245, 1.8169) (68.0248, 1.8169) knots 0 0 0 1 2 2 2
  spline S126 degree 2 poles (78.4462, 5.7472) (78.4462, 3.851) (76.6229, 1.7845) (75.0994, 1.7845) knots 0 0 0 1 2 2 2
  spline S127 degree 2 poles (75.0994, 1.7845) (73.5353, 1.7845) (71.7444, 3.9158) (71.7444, 5.7472) knots 0 0 0 1 2 2 2
  spline S128 degree 2 poles (71.7444, 5.7472) (71.7444, 7.6273) (73.5921, 9.71) (75.0994, 9.71) knots 0 0 0 1 2 2 2
  spline S129 degree 2 poles (75.0994, 9.71) (76.6229, 9.71) (78.4462, 7.6354) (78.4462, 5.7472) knots 0 0 0 1 2 2 2
  spline S130 degree 2 poles (77.1415, 5.7472) (77.1415, 7.2059) (76.0799, 8.6241) (75.0994, 8.6241) knots 0 0 0 1 2 2 2
  spline S131 degree 2 poles (75.0994, 8.6241) (74.1188, 8.6241) (73.0491, 7.2059) (73.0491, 5.7472) knots 0 0 0 1 2 2 2
  spline S132 degree 2 poles (73.0491, 5.7472) (73.0491, 4.3291) (74.1188, 2.8704) (75.0994, 2.8704) knots 0 0 0 1 2 2 2
  spline S133 degree 2 poles (75.0994, 2.8704) (76.0718, 2.8704) (77.1415, 4.3048) (77.1415, 5.7472) knots 0 0 0 1 2 2 2
  line L157 (85.6342, 1.9952) -> (84.37, 1.9952)
  line L158 (84.37, 1.9952) -> (84.37, 6.274)
  spline S134 degree 2 poles (84.37, 6.274) (84.37, 6.7926) (84.2728, 7.684) (84.1269, 7.9515) knots 0 0 0 1 2 2 2
  spline S135 degree 2 poles (84.1269, 7.9515) (83.9729, 8.2351) (83.4219, 8.5106) (82.9519, 8.5106) knots 0 0 0 1 2 2 2
  spline S136 degree 2 poles (82.9519, 8.5106) (82.4818, 8.5106) (81.4851, 8.0082) (81.007, 7.603) knots 0 0 0 1 2 2 2
  line L159 (81.007, 7.603) -> (81.007, 1.9952)
  line L160 (81.007, 1.9952) -> (79.7428, 1.9952)
  line L161 (79.7428, 1.9952) -> (79.7428, 9.4993)
  line L162 (79.7428, 9.4993) -> (81.007, 9.4993)
  line L163 (81.007, 9.4993) -> (81.007, 8.6646)
  spline S137 degree 2 poles (81.007, 8.6646) (81.5742, 9.1751) (82.6682, 9.71) (83.2841, 9.71) knots 0 0 0 1 2 2 2
  spline S138 degree 2 poles (83.2841, 9.71) (84.3862, 9.71) (85.6342, 8.2513) (85.6342, 6.8656) knots 0 0 0 1 2 2 2
  line L164 (85.6342, 6.8656) -> (85.6342, 1.9952)
  spline S139 degree 2 poles (89.678, 1.8493) (88.6488, 1.8493) (87.49, 3.0244) (87.49, 4.2967) knots 0 0 0 1 2 2 2
  line L165 (87.49, 4.2967) -> (87.49, 8.4539)
  line L166 (87.49, 8.4539) -> (86.6391, 8.4539)
  line L167 (86.6391, 8.4539) -> (86.6391, 9.4993)
  line L168 (86.6391, 9.4993) -> (87.49, 9.4993)
  line L169 (87.49, 9.4993) -> (87.49, 11.6549)
  line L170 (87.49, 11.6549) -> (88.7541, 11.6549)
  line L171 (88.7541, 11.6549) -> (88.7541, 9.4993)
  line L172 (88.7541, 9.4993) -> (91.0799, 9.4993)
  line L173 (91.0799, 9.4993) -> (91.0799, 8.4539)
  line L174 (91.0799, 8.4539) -> (88.7541, 8.4539)
  line L175 (88.7541, 8.4539) -> (88.7541, 4.8801)
  spline S140 degree 2 poles (88.7541, 4.8801) (88.7541, 4.3129) (88.7947, 3.6889) (88.9324, 3.4215) knots 0 0 0 1 2 2 2
  spline S141 degree 2 poles (88.9324, 3.4215) (89.0459, 3.1865) (89.5564, 2.9515) (89.994, 2.9515) knots 0 0 0 1 2 2 2
  spline S142 degree 2 poles (89.994, 2.9515) (90.3019, 2.9515) (90.8773, 3.1378) (91.007, 3.1946) knots 0 0 0 1 2 2 2
  line L176 (91.007, 3.1946) -> (91.0799, 3.1946)
  line L177 (91.0799, 3.1946) -> (91.0799, 2.06)
  spline S143 degree 2 poles (91.0799, 2.06) (90.7233, 1.9628) (89.994, 1.8493) (89.678, 1.8493) knots 0 0 0 1 2 2 2
  line L178 (95.9908, 8.1459) -> (95.9259, 8.1459)
  spline S144 degree 2 poles (95.9259, 8.1459) (95.7801, 8.1865) (95.464, 8.2027) (95.2452, 8.2027) knots 0 0 0 1 2 2 2
  spline S145 degree 2 poles (95.2452, 8.2027) (94.7347, 8.2027) (93.7298, 7.757) (93.276, 7.3194) knots 0 0 0 1 2 2 2
  line L179 (93.276, 7.3194) -> (93.276, 1.9952)
  line L180 (93.276, 1.9952) -> (92.0118, 1.9952)
  line L181 (92.0118, 1.9952) -> (92.0118, 9.4993)
  line L182 (92.0118, 9.4993) -> (93.276, 9.4993)
  line L183 (93.276, 9.4993) -> (93.276, 8.381)
  spline S146 degree 2 poles (93.276, 8.381) (93.9648, 8.9968) (94.994, 9.4993) (95.4802, 9.4993) knots 0 0 0 1 2 2 2
  spline S147 degree 2 poles (95.4802, 9.4993) (95.6747, 9.4993) (95.8692, 9.4831) (95.9908, 9.4587) knots 0 0 0 1 2 2 2
  line L184 (95.9908, 9.4587) -> (95.9908, 8.1459)
  spline S148 degree 2 poles (103.1382, 5.7472) (103.1382, 3.851) (101.3149, 1.7845) (99.7914, 1.7845) knots 0 0 0 1 2 2 2
  spline S149 degree 2 poles (99.7914, 1.7845) (98.2274, 1.7845) (96.4365, 3.9158) (96.4365, 5.7472) knots 0 0 0 1 2 2 2
  spline S150 degree 2 poles (96.4365, 5.7472) (96.4365, 7.6273) (98.2841, 9.71) (99.7914, 9.71) knots 0 0 0 1 2 2 2
  spline S151 degree 2 poles (99.7914, 9.71) (101.3149, 9.71) (103.1382, 7.6354) (103.1382, 5.7472) knots 0 0 0 1 2 2 2
  spline S152 degree 2 poles (101.8335, 5.7472) (101.8335, 7.2059) (100.772, 8.6241) (99.7914, 8.6241) knots 0 0 0 1 2 2 2
  spline S153 degree 2 poles (99.7914, 8.6241) (98.8109, 8.6241) (97.7412, 7.2059) (97.7412, 5.7472) knots 0 0 0 1 2 2 2
  spline S154 degree 2 poles (97.7412, 5.7472) (97.7412, 4.3291) (98.8109, 2.8704) (99.7914, 2.8704) knots 0 0 0 1 2 2 2
  spline S155 degree 2 poles (99.7914, 2.8704) (100.7639, 2.8704) (101.8335, 4.3048) (101.8335, 5.7472) knots 0 0 0 1 2 2 2
  line L185 (105.7233, 1.9952) -> (104.4592, 1.9952)
  line L186 (104.4592, 1.9952) -> (104.4592, 12.4409)
  line L187 (104.4592, 12.4409) -> (105.7233, 12.4409)
  line L188 (105.7233, 12.4409) -> (105.7233, 1.9952)
  line L189 (108.8676, 1.9952) -> (107.6034, 1.9952)
  line L190 (107.6034, 1.9952) -> (107.6034, 12.4409)
  line L191 (107.6034, 12.4409) -> (108.8676, 12.4409)
  line L192 (108.8676, 12.4409) -> (108.8676, 1.9952)
  spline S156 degree 2 poles (113.981, 1.825) (112.182, 1.825) (110.2047, 3.8429) (110.2047, 5.7067) knots 0 0 0 1 2 2 2
  spline S157 degree 2 poles (110.2047, 5.7067) (110.2047, 7.5382) (112.1253, 9.71) (113.6731, 9.71) knots 0 0 0 1 2 2 2
  spline S158 degree 2 poles (113.6731, 9.71) (114.37, 9.71) (115.4478, 9.3048) (115.8449, 8.8753) knots 0 0 0 1 2 2 2
  spline S159 degree 2 poles (115.8449, 8.8753) (116.2501, 8.4458) (116.6796, 7.2059) (116.6796, 6.3064) knots 0 0 0 1 2 2 2
  line L193 (116.6796, 6.3064) -> (116.6796, 5.6176)
  line L194 (116.6796, 5.6176) -> (111.4851, 5.6176)
  spline S160 degree 2 poles (111.4851, 5.6176) (111.4851, 4.3129) (112.7979, 2.9271) (113.9648, 2.9271) knots 0 0 0 1 2 2 2
  spline S161 degree 2 poles (113.9648, 2.9271) (114.3781, 2.9271) (115.1804, 3.1135) (115.5045, 3.2594) knots 0 0 0 1 2 2 2
  spline S162 degree 2 poles (115.5045, 3.2594) (115.8449, 3.4215) (116.3149, 3.7051) (116.4689, 3.8348) knots 0 0 0 1 2 2 2
  line L195 (116.4689, 3.8348) -> (116.5418, 3.8348)
  line L196 (116.5418, 3.8348) -> (116.5418, 2.4571)
  spline S163 degree 2 poles (116.5418, 2.4571) (116.323, 2.368) (115.6585, 2.1087) (115.3992, 2.0357) knots 0 0 0 1 2 2 2
  spline S164 degree 2 poles (115.3992, 2.0357) (115.0345, 1.9304) (114.4348, 1.825) (113.981, 1.825) knots 0 0 0 1 2 2 2
  spline S165 degree 2 poles (115.4478, 6.5819) (115.4316, 7.0925) (115.2209, 7.838) (115.0183, 8.0892) knots 0 0 0 1 2 2 2
  spline S166 degree 2 poles (115.0183, 8.0892) (114.7995, 8.3728) (114.1107, 8.6727) (113.6002, 8.6727) knots 0 0 0 1 2 2 2
  spline S167 degree 2 poles (113.6002, 8.6727) (113.0977, 8.6727) (112.3927, 8.3728) (112.101, 8.0811) knots 0 0 0 1 2 2 2
  spline S168 degree 2 poles (112.101, 8.0811) (111.8173, 7.7813) (111.5256, 7.06) (111.4851, 6.5819) knots 0 0 0 1 2 2 2
  line L197 (111.4851, 6.5819) -> (115.4478, 6.5819)
  line L198 (121.9389, 8.1459) -> (121.8741, 8.1459)
  spline S169 degree 2 poles (121.8741, 8.1459) (121.7282, 8.1865) (121.4122, 8.2027) (121.1934, 8.2027) knots 0 0 0 1 2 2 2
  spline S170 degree 2 poles (121.1934, 8.2027) (120.6828, 8.2027) (119.678, 7.757) (119.2241, 7.3194) knots 0 0 0 1 2 2 2
  line L199 (119.2241, 7.3194) -> (119.2241, 1.9952)
  line L200 (119.2241, 1.9952) -> (117.96, 1.9952)
  line L201 (117.96, 1.9952) -> (117.96, 9.4993)
  line L202 (117.96, 9.4993) -> (119.2241, 9.4993)
  line L203 (119.2241, 9.4993) -> (119.2241, 8.381)
  spline S171 degree 2 poles (119.2241, 8.381) (119.913, 8.9968) (120.9421, 9.4993) (121.4284, 9.4993) knots 0 0 0 1 2 2 2
  spline S172 degree 2 poles (121.4284, 9.4993) (121.6229, 9.4993) (121.8173, 9.4831) (121.9389, 9.4587) knots 0 0 0 1 2 2 2
  line L204 (121.9389, 9.4587) -> (121.9389, 8.1459)
  point P0 (142.4317, -0.2259)
  constraints: 6 other
extrude "Extrusion2" add sketch "Sketch2" against normal blind 2
ref_plane "Work Plane3" through (-0.0003, -144.9621, -142.4319) normal (0, 0, -1) x (-1, 0, 0)